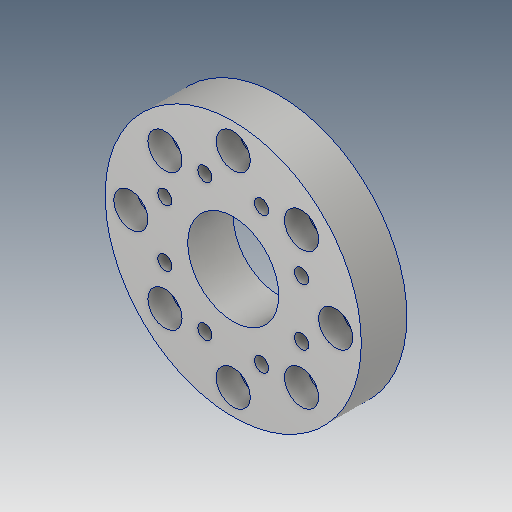
# Autodesk Inventor part: 조인트1고관절축
Saved by Autodesk Inventor 2020.5 (Build 245400000, 400)
## iProperties
Created: 2021-07-19
Part Number: 조인트1고관절축
Material: 알루미늄 6061
Document SubType Name: Modeling
Designer: user
Density: 2.7 g/cm^3
Appearance: 알루미늄 - 평지
Mass: 26.0244 g
Surface Area: 55.3216 cm^2
Volume: 9.63866 cm^3
Author: user
Autodesk Inventor part; units mm, degrees
ref_plane "YZ Plane" through (0, 0, 0) normal (1, 0, 0) x (0, 1, 0)
ref_plane "XZ Plane" through (0, 0, 0) normal (0, 1, 0) x (-1, 0, 0)
ref_plane "XY Plane" through (0, 0, 0) normal (0, 0, 1) x (1, 0, 0)
sketch "스케치1" plane through (0, 0, 0) normal (0, 0, 1) x (1, 0, 0)
  circle A0 centre (0, 0) radius 22.5
  dimension "d0" = 45
  constraints: 1 centre point, 1 coincident
  measures "d0" diameter of A0
extrude "돌출1" add sketch "스케치1" along normal blind 8
sketch "스케치2" plane through (0, 0, 8) normal (0, 0, 1) x (1, 0, 0)
  circle A0 centre (0, 0) radius 8
  dimension "d3" = 16
  constraints: 1 centre point, 1 coincident
  measures "d3" diameter of A0
extrude "돌출2" cut sketch "스케치2" against normal up to surface (8 mm away)
sketch "스케치3" plane through (0, 0, 8) normal (0, 0, 1) x (1, 0, 0)
  line L0 (-0.15, -20.7995) -> (-0.15, -19.593)
  arc A0 (-0.15, -16.407) -> (-0.15, -19.593) centre (0, -18) ccw
  line L1 (-0.15, -16.407) -> (-0.15, -12.9991)
  arc A1 (0.15, -12.9991) -> (-0.15, -12.9991) centre (0, 0) ccw
  line L2 (0.15, -16.407) -> (0.15, -12.9991)
  arc A2 (0.15, -19.593) -> (0.15, -16.407) centre (0, -18) ccw
  line L3 (0.15, -20.7995) -> (0.15, -19.593)
  arc A3 (0.15, -20.7995) -> (-0.15, -20.7995) centre (0, 0) ccw
  circle A4 centre (12, 12) radius 1.6
  circle A5 centre (-18, 0) radius 1.6
  circle A6 centre (-12, 12) radius 1.6
  circle A7 centre (-12, -12) radius 1.6
  circle A8 centre (18, 0) radius 1.6
  circle A9 centre (12, -12) radius 1.6
  circle A10 centre (6, 18) radius 1
  circle A11 centre (-6, 18) radius 1
  circle A12 centre (-18, 6) radius 1
  circle A13 centre (-18, -6) radius 1
  circle A14 centre (-6, -18) radius 1
  circle A15 centre (6, -18) radius 1
  circle A16 centre (18, -6) radius 1
  circle A17 centre (18, 6) radius 1
  circle A18 centre (0, 18) radius 1.6
  circle A19 centre (0, 0) radius 12.5
  line L4 (-27, -21) -> (-21, -21)
  line L5 (-21, -21) -> (-21, -27)
  line L6 (25, -27) -> (27, -25)
  line L7 (27, -25) -> (27, 25)
  line L8 (27, 25) -> (25, 27)
  line L9 (25, 27) -> (-25, 27)
  line L10 (-25, 27) -> (-27, 25)
  line L11 (-27, 25) -> (-27, -25)
  line L12 (-27, -25) -> (-25, -27)
  line L13 (-25, -27) -> (25, -27)
  circle A20 centre (0, 0) radius 26.75
  circle A21 centre (24, -24) radius 1.6
  circle A22 centre (-24, -24) radius 1.6
  circle A23 centre (24, 24) radius 1.6
  circle A24 centre (-24, 24) radius 1.6
  circle A25 centre (0, -18) radius 1.6
  dimension "d6" = 3.2
  constraints: 28 end point, 26 centre point, 8 point on circle, 1 coincident
  measures "d6" diameter of A25
extrude "돌출3" cut sketch "스케치3" against normal up to surface (8 mm away) contours A0 A25 A2 | A4 | A5 | A6 | A7 | A8 | A9 | A18
sketch "스케치4" plane through (0, 0, 8) normal (0, 0, 1) x (1, 0, 0)
  circle A0 centre (0, 18) radius 1.6 projected
  circle A1 centre (-18, 0) radius 1.6 projected
  circle A2 centre (-12, -12) radius 1.6 projected
  circle A3 centre (12, 12) radius 1.6 projected
  circle A4 centre (18, 0) radius 1.6 projected
  circle A5 centre (0, -18) radius 1.6 projected
  circle A6 centre (12, -12) radius 1.6 projected
  circle A7 centre (-12, 12) radius 1.6 projected
  circle A8 centre (0, 0) radius 8 projected
  circle A9 centre (0, 0) radius 22.5 projected
  circle A10 centre (-18, 0) radius 3
  circle A11 centre (-12, 12) radius 3
  circle A12 centre (0, 18) radius 1.6 projected
  circle A13 centre (0, 18) radius 3
  circle A14 centre (12, 12) radius 1.6 projected
  circle A15 centre (12, 12) radius 3
  circle A16 centre (18, 0) radius 3
  circle A17 centre (12, -12) radius 1.6 projected
  circle A18 centre (12, -12) radius 3
  circle A19 centre (0, -18) radius 3
  circle A20 centre (-12, -12) radius 3
  dimension "d9" = 6
  dimension "d10" = 6
  dimension "d11" = 6
  dimension "d12" = 6
  dimension "d13" = 6
  dimension "d14" = 6
  dimension "d15" = 6
  dimension "d16" = 6
  constraints: 8 centre point, 8 coincident
  measures "d9" diameter of A10
  measures "d10" diameter of A11
  measures "d11" diameter of A13
  measures "d12" diameter of A15
  measures "d13" diameter of A16
  measures "d14" diameter of A18
  measures "d15" diameter of A19
  measures "d16" diameter of A20
extrude "돌출4" cut sketch "스케치4" against normal blind 4 contours A10 | A11 | A13 | A15 | A16 | A18 | A19 | A20
sketch "스케치5" plane through (0, 0, 8) normal (0, 0, 1) x (1, 0, 0)
  line L0 (0, 0) -> (12.0104, 4.9749)
  line L1 (0, 0) -> (13, 0) construction
  circle A0 centre (12.0104, 4.9749) radius 1.25
  circle A1 centre (4.9749, 12.0104) radius 1.25
  circle A2 centre (-4.9749, 12.0104) radius 1.25
  circle A3 centre (-12.0104, 4.9749) radius 1.25
  circle A4 centre (-12.0104, -4.9749) radius 1.25
  circle A5 centre (-4.9749, -12.0104) radius 1.25
  circle A6 centre (4.9749, -12.0104) radius 1.25
  circle A7 centre (12.0104, -4.9749) radius 1.25
  dimension "d19" = 13
  dimension "d20" = 22.5
  dimension "d21" = 2.5
  dimension "d24" = 360
  constraints: 8 centre point, 4 end point, 1 coincident, 1 equal length, 1 horizontal, 17 other
  measures "d19" distance of L0.start L0.end
  measures "d20" angle of L1 L0
  measures "d21" diameter of A0
extrude "돌출5" cut sketch "스케치5" against normal up to surface (8 mm away)
equation "\"d4\" = d3"
